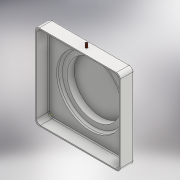
# Autodesk Inventor part: Hot Plate
Saved by Autodesk Inventor 2020 (Build 240168000, 168)
## iProperties
Created: 2018-04-19
Part Number: Hot Plate
Material: Generic
Document SubType Name: Modeling
Designer: PC  USER
Density: 1 g/cm^3
Appearance: Default
Author: PC  USER
Autodesk Inventor part; units mm, degrees
ref_plane "YZ Plane" through (0, 0, 0) normal (1, 0, 0) x (0, 1, 0)
ref_plane "XZ Plane" through (0, 0, 0) normal (0, 1, 0) x (-1, 0, 0)
ref_plane "XY Plane" through (0, 0, 0) normal (0, 0, 1) x (1, 0, 0)
sketch "Sketch1" plane through (0, 0, 0) normal (0, 1, 0) x (-1, 0, 0)
  line L0 (110, 110) -> (-110, 110)
  line L1 (-110, 110) -> (-110, -110)
  line L2 (-110, -110) -> (110, -110)
  line L3 (110, -110) -> (110, 110)
  point P0 (0, 0)
  point P1 (110, 0)
  point P2 (0, -110)
  dimension "d0" = 220
  constraints: 8 end point, 2 midpoint, 2 parallel, 2 perpendicular, 1 horizontal, 1 horizontal alignment, 1 vertical alignment
  measures "d0" distance of L1.end L2.end
extrude "Extrusion1" add sketch "Sketch1" along normal blind 35
sketch "Sketch2" plane through (0, 35, 0) normal (0, 1, 0) x (1, 0, 0)
  circle A0 centre (0, 0) radius 90
  dimension "d3" = 180
  constraints: 1 centre point, 1 coincident
  measures "d3" diameter of A0
extrude "Extrusion2" add sketch "Sketch2" along normal blind 10
sketch "Sketch3" plane through (0, 45, 0) normal (0, 1, 0) x (1, 0, 0)
  circle A0 centre (0, 0) radius 72.5
  dimension "d6" = 145
  constraints: 1 centre point, 1 coincident
  measures "d6" diameter of A0
extrude "Extrusion3" add sketch "Sketch3" along normal blind 18
sketch "Sketch4" plane through (-110, 0, 110) normal (0, 0, 1) x (1, 0, 0)
  circle A0 centre (115, 17.5) radius 3
  line L0 (220, 0) -> (220, 35) projected
  circle A1 centre (115, 17.5) radius 2.5
  point P0 (110, 0)
  dimension "d9" = 6
  dimension "d10" = 105
  dimension "d11" = 17.5
  dimension "d33" = 0.5
  dimension "d34" = 5
  constraints: 2 centre point
  measures "d9" diameter of A0
  measures "d10" distance from line of L0 A0.centre
  measures "d11" vertical distance of point (110, 0) A0.centre
  measures "d33" radial gap between concentric circles of A0 A1
  measures "d34" diameter of A1
shell "Shell1" thickness 3 removed faces 1 at (36.6667, 0, 36.6667)
fillet "Fillet1" radius 10 4 edges at (110, 17.5, 110) (-110, 17.5, 110) (110, 17.5, -110) (-110, 17.5, -110)
fillet "Fillet1" radius 2.5 4 edges at (0, 35, 110) (0, 35, -110) (-110, 35, 0) (110, 35, 0)
fillet "Fillet1" radius 5 1 edges at (-90, 45, 0)
fillet "Fillet3" radius 8 1 edges at (-90, 35, 0)
fillet "Fillet4" radius 10 4 edges at (-107, 16, -107) (-107, 16, 107) (107, 16, 107) (107, 16, -107)
fillet "Fillet4" radius 2.5 4 edges at (-107, 32, 0) (0, 32, 107) (107, 32, 0) (0, 32, -107)
fillet "Fillet4" radius 5 1 edges at (-87, 42, 0)
sketch "Sketch5" plane through (0, 63, 0) normal (0, 1, 0) x (1, 0, 0)
  circle A0 centre (0, 0) radius 137.5 construction
  line L0 (0, 0) -> (114.1894, -114.1894) construction
  line L1 (0, 0) -> (161.4882, 0) construction
  line L2 (114.1894, -114.1894) -> (-122.4575, 122.4575) construction
  line L3 (118.52, 118.52) -> (-114.1894, -114.1894) construction
  circle A1 centre (97.2272, -97.2272) radius 0.5
  dimension "d23" = 275
  dimension "d24" = 45
  dimension "d25" = 1
  constraints: 8 end point, 2 point on line, 1 centre point, 1 coincident, 1 equal length, 1 horizontal, 3 other
  measures "d24" angle of L0 L1
  measures "d25" diameter of A1
extrude "Extrusion5" cut sketch "Sketch5" against normal through all
pattern_circular "Circular Pattern1" count 4 over 360 about axis through (0, -10, 0) along (0, 1, 0) of "Extrusion5"
extrude "Extrusion6" add sketch "Sketch4" along normal blind 10
body "Solid1"
